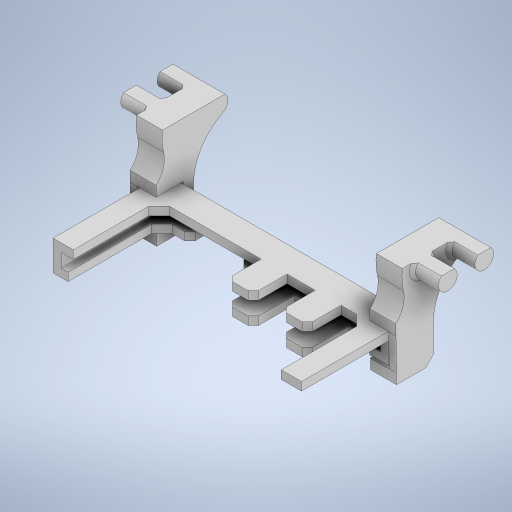
# Autodesk Inventor part: Holder-PCB
Saved by Autodesk Inventor 2024.3 (Build 283343000, 343)
## iProperties
Created: 2025-01-23
Part Number: Holder-PCB
Material: Generic
Document SubType Name: Modeling
Designer: ASUS TUF
Density: 1 g/cm^3
Appearance: Default
Author: ASUS TUF
Autodesk Inventor part; units mm, degrees
ref_plane "YZ Plane" through (0, 0, 0) normal (1, 0, 0) x (0, 1, 0)
ref_plane "XZ Plane" through (0, 0, 0) normal (0, 1, 0) x (-1, 0, 0)
ref_plane "XY Plane" through (0, 0, 0) normal (0, 0, 1) x (1, 0, 0)
sketch "Sketch1" plane through (0, 0, 0) normal (0, 0, 1) x (1, 0, 0)
  line L0 (22, 1) -> (22, -1) construction
  line L1 (-22, -1) -> (22, -1) construction
  line L2 (-22, 1) -> (-22, -1) construction
  line L3 (22, 1) -> (-22, 1) construction
  line L4 (22.3, -1.3) -> (22.3, 1.3)
  line L5 (22.3, 1.3) -> (-22.3, 1.3)
  line L6 (-22.3, 1.3) -> (-22.3, -1.3)
  line L7 (-22.3, -1.3) -> (22.3, -1.3)
  line L8 (-20, -1) -> (-20, -4.5) construction
  line L9 (23.9, -2.9) -> (23.9, 2.9)
  line L10 (23.9, 2.9) -> (-23.9, 2.9)
  line L11 (-23.9, 2.9) -> (-23.9, -2.9)
  line L12 (-23.9, -2.9) -> (23.9, -2.9)
  line L13 (-21, -2.9) -> (-21, 2.9)
  line L14 (0, -2.9) -> (0, 2.9) construction
  line L15 (21, -2.9) -> (21, 2.9)
  point P0 (0, 0)
  point P1 (21, -1.3)
  point P2 (21, 1.3)
  point P3 (-21, 1.3)
  point P4 (-21, -1.3)
  dimension "d2" = 0.3
  dimension "d3" = 1.6
  dimension "d4" = 1
  constraints: 22 end point, 2 midpoint, 2 point on line, 2 symmetric about line, 1 perpendicular, 6 other
  measures "d2" distance between parallel lines of L1 L7
  measures "d3" distance between parallel lines of L7 L12
  measures "d4" distance between parallel lines of L8 L13
extrude "Extrusion1" add sketch "Sketch1" along normal mid plane 1.5
sketch "Sketch2" plane through (0, 0, 0.75) normal (0, 0, 1) x (1, 0, 0)
  line L0 (22, 1) -> (22, -1) construction
  line L1 (-22, -1) -> (22, -1) construction
  line L2 (-22, 1) -> (-22, -1) construction
  line L3 (22, 1) -> (-22, 1) construction
  line L4 (-20, -1) -> (-20, -4.5) construction
  line L5 (23.9, -2.9) -> (-23.9, -2.9) projected
  line L6 (-23.9, -2.9) -> (-23.9, 2.9) projected
  line L7 (-23.9, 2.9) -> (23.9, 2.9) projected
  line L8 (23.9, 2.9) -> (23.9, -2.9) projected
  line L9 (22.3, -1.3) -> (22.3, 1.3)
  line L10 (22.3, 1.3) -> (-22.3, 1.3)
  line L11 (-22.3, 1.3) -> (-22.3, -1.3)
  line L12 (-22.3, -1.3) -> (22.3, -1.3)
  line L13 (-21, -2.9) -> (-21, -1.3)
  line L14 (0, -2.9) -> (0, 2.9) construction
  line L15 (-20, 1.3) -> (-20, 2.9)
  line L16 (21, -2.9) -> (21, -1.3)
  line L17 (20, 1.3) -> (20, 2.9)
  point P0 (0, 0)
  point P1 (-21, 1.3)
  dimension "d5" = 0.3
  dimension "d6" = 1
  dimension "d9" = 2
  constraints: 18 end point, 4 point on line, 4 symmetric about line, 2 midpoint, 2 perpendicular, 3 other
  measures "d5" distance between parallel lines of L1 L12
  measures "d6" distance between parallel lines of L4 L13
  measures "d9" distance between parallel lines of L2 L15
extrude "Extrusion2" add sketch "Sketch2" along normal blind 20 contours L5 L16 L12 L9 L10 L17 L7 L8 | L5 L6 L7 L15 L10 L11 L12 L13
sketch "Sketch3" plane through (0, 0, 0.75) normal (0, 0, 1) x (1, 0, 0)
  line L0 (-20, 2.9) -> (-20, 1.3)
  line L1 (-20, 1.3) -> (-22.3, 1.3)
  line L2 (-22.3, 1.3) -> (-22.3, -1.3)
  line L3 (-22.3, -1.3) -> (-21, -1.3)
  line L4 (-21, -1.3) -> (-21, -2.9)
  line L5 (-21, -2.9) -> (21, -2.9)
  line L6 (21, -2.9) -> (21, -1.3)
  line L7 (21, -1.3) -> (22.3, -1.3)
  line L8 (22.3, -1.3) -> (22.3, 1.3)
  line L9 (22.3, 1.3) -> (20, 1.3)
  line L10 (20, 1.3) -> (20, 2.9)
  line L11 (20, 2.9) -> (-20, 2.9)
  line L12 (-20, 1.3) -> (20, 1.3)
  line L13 (21, -1.3) -> (-21, -1.3)
  line L14 (-0.881943, -1.696277) -> (-0.881943, -10.1) construction
  line L15 (5.118057, -10.8) -> (5.118057, -1) construction
  line L16 (-0.381943, -2.9) -> (-0.381943, 2.9)
  line L17 (4.618057, 2.9) -> (4.618057, -2.9)
  line L18 (20, 2.9) -> (-20, 2.9)
  line L19 (9.518057, -1.696277) -> (9.518057, -10.1) construction
  line L20 (15.518057, -0.5) -> (15.518057, -6.5) construction
  line L21 (10.018057, 2.9) -> (10.018057, -2.9)
  line L22 (-21, -2.9) -> (21, -2.9)
  line L23 (15.018057, 2.9) -> (15.018057, -2.9)
  point P0 (0, 0)
  point P1 (15.018057, 1.3)
  point P2 (10.018057, 1.3)
  point P3 (4.618057, 1.3)
  point P4 (-0.381943, 1.3)
  point P5 (15.018057, -1.3)
  point P6 (10.018057, -1.3)
  point P7 (4.618057, -1.3)
  point P8 (-0.381943, -1.3)
  dimension "d21" = 0.5
  dimension "d22" = 0.5
  dimension "d23" = 0.5
  dimension "d24" = 0.5
  constraints: 20 end point, 8 point on line, 5 perpendicular, 4 vertical, 1 horizontal, 1 parallel, 8 other
  measures "d21" distance between parallel lines of L14 L16
  measures "d22" distance between parallel lines of L15 L17
  measures "d23" distance between parallel lines of L20 L23
  measures "d24" distance between parallel lines of L19 L21
extrude "Extrusion3" add sketch "Sketch3" along normal blind 3.5 contours L11 L16 L12 L0 | L11 L17 L12 L16 | L11 L21 L12 L17 | L11 L23 L12 L21 | L11 L10 L12 L23
extrude "Extrusion4" add sketch "Sketch3" along normal blind 2 contours L16 L5 L4 L13 | L13 L17 L5 L16 | L13 L21 L5 L17 | L13 L23 L5 L21 | L13 L6 L5 L23
chamfer "Chamfer1" distance 2 angle 45 4 edges at (-21, -2.1, 2.75) (-20, 2.1, 4.25) (20, 2.1, 4.25) (21, -2.1, 2.75)
sketch "Sketch4" plane through (-23.9, -2.9, -0.75) normal (0, -1, 0) x (1, 0, 0)
  line L0 (9.318057, -1.3) -> (11.268057, -1.3) construction
  line L1 (11.268057, -1.3) -> (11.268057, 2.4) construction
  line L2 (11.268057, 2.4) -> (14.768057, 2.4) construction
  line L3 (14.768057, 2.4) -> (14.768057, -1.3) construction
  line L4 (14.768057, -1.3) -> (16.718057, -1.3) construction
  line L5 (16.718057, -1.3) -> (16.718057, 6) construction
  line L6 (16.718057, 6) -> (9.318057, 6) construction
  line L7 (9.318057, 6) -> (9.318057, -1.3) construction
  line L8 (46.718057, 5.7) -> (46.718057, 7.65) construction
  line L9 (46.718057, 7.65) -> (43.018057, 7.65) construction
  line L10 (43.018057, 7.65) -> (43.018057, 11.15) construction
  line L11 (43.018057, 11.15) -> (46.718057, 11.15) construction
  line L12 (46.718057, 11.15) -> (46.718057, 13.1) construction
  line L13 (46.718057, 13.1) -> (39.418057, 13.1) construction
  line L14 (39.418057, 13.1) -> (39.418057, 5.7) construction
  line L15 (39.418057, 5.7) -> (46.718057, 5.7) construction
  line L16 (17.718057, 7) -> (17.718057, -2.3)
  line L17 (17.718057, -2.3) -> (13.768057, -2.3)
  line L18 (13.768057, -2.3) -> (13.768057, 1.4)
  line L19 (13.768057, 1.4) -> (12.268057, 1.4)
  line L20 (12.268057, 1.4) -> (12.268057, -2.3)
  line L21 (12.268057, -2.3) -> (8.318057, -2.3)
  line L22 (8.318057, -2.3) -> (8.318057, 7)
  line L23 (8.318057, 7) -> (17.718057, 7)
  line L24 (47.718057, 4.7) -> (47.718057, 8.65)
  line L25 (47.718057, 8.65) -> (44.018057, 8.65)
  line L26 (44.018057, 8.65) -> (44.018057, 10.15)
  line L27 (44.018057, 10.15) -> (47.718057, 10.15)
  line L28 (47.718057, 10.15) -> (47.718057, 14.1)
  line L29 (47.718057, 14.1) -> (38.418057, 14.1)
  line L30 (38.418057, 14.1) -> (38.418057, 4.7)
  line L31 (38.418057, 4.7) -> (47.718057, 4.7)
  line L32 (47.8, 0) -> (47.8, 21.5)
  line L33 (44.9, 21.5) -> (47.8, 21.5)
  line L34 (44.9, 5.5) -> (44.9, 21.5)
  line L35 (42.9, 3.5) -> (44.9, 5.5)
  line L36 (4.9, 3.5) -> (42.9, 3.5)
  line L37 (2.9, 5.5) -> (4.9, 3.5)
  line L38 (2.9, 5.5) -> (2.9, 21.5)
  line L39 (0, 21.5) -> (2.9, 21.5)
  line L40 (0, 21.5) -> (0, 0)
  line L41 (47.8, 0) -> (0, 0)
  line L42 (47.718057, 4.7) -> (47.8, 4.7)
  line L43 (47.718057, 14.1) -> (47.8, 14.1)
  point P0 (23.9, 0.75)
  point P1 (17.718057, 0)
  point P2 (17.718057, 3.5)
  point P3 (8.318057, 3.5)
  point P4 (8.318057, 0)
  point P5 (44.9, 14.1)
  point P6 (44.1, 4.7)
  dimension "d17" = 1
  dimension "d18" = 1
  constraints: 36 end point, 2 perpendicular, 2 point on line, 14 other
  measures "d17" distance between parallel lines of L5 L16
  measures "d18" distance between parallel lines of L15 L31
extrude "Extrusion5" cut sketch "Sketch4" against normal up to surface (4.2 mm away) contours L16 L41 L18 L19 L20 L22 L36 | L41 L20 L19 L18 | L35 L34 L25 L24 L31 | L42 L24 L25 L34 L27 L28 L43 L32 | L43 L29 L34 L33 L32 | L28 L27 L34 L29
extrude "Extrusion6" add sketch "Sketch3" along normal blind 8 from surface at 2 contours L11 L17 L12 L16 | L13 L17 L5 L16 | L11 L23 L12 L21 | L13 L23 L5 L21
chamfer "Chamfer2" distance 1 angle 45 10 edges at (4.6181, 2.1, 10.75) (4.6181, -2.1, 10.75) (-0.3819, 2.1, 10.75) (-0.3819, -2.1, 10.75) (10.0181, 2.1, 10.75) (10.0181, -2.1, 10.75) (15.0181, 2.1, 10.75) (15.0181, -2.1, 10.75) (-6.1819, -2.1, 2.75) (-15.5819, -2.1, 2.75)
ref_plane "Work Plane1" through (25.567949, 17.21409, -10.739318) normal (-1, 0, 0) x (0, 0, -1)
sketch "Sketch5" plane through (25.567949, 17.21409, -10.739318) normal (-1, 0, 0) x (0, 0, -1)
  arc A0 (-1.677124, 3.328427) -> (-4.322876, 3.328427) centre (-3, 4.828427) ccw
  line L0 (-1.677124, 3.328427) -> (-4.322876, 3.328427)
  arc A1 (-9.608071, 10.950914) -> (-8.094331, 12.258046) centre (-9.829369, 12.737259) ccw
  arc A2 (-7.504205, 12.629939) -> (-8.094331, 12.258046) centre (-3, 4.828427) ccw
  arc A3 (-5.970033, 8.970542) -> (-7.504205, 12.629939) centre (-6.504205, 10.897888) ccw
  arc A4 (-5.970033, 8.970542) -> (-6.678281, 8.227605) centre (-5.702948, 8.006869) ccw
  arc A5 (-6.678281, 8.227605) -> (-7.782915, 6.314323) centre (-3, 4.828427) ccw
  arc A6 (-7.782915, 6.314323) -> (-8.072193, 5.329494) centre (-7.104086, 5.580027) ccw
  arc A7 (-8.685534, 3.328427) -> (-8.072193, 5.329494) centre (-10.008409, 4.828427) ccw
  line L1 (-8.685534, 3.328427) -> (-11.331285, 3.328427)
  arc A8 (-11.721843, 5.860001) -> (-11.331285, 3.328427) centre (-10.008409, 4.828427) ccw
  arc A9 (-11.721843, 5.860001) -> (-11.606264, 7.489941) centre (-13.263933, 6.788418) ccw
  arc A10 (-9.608071, 10.950914) -> (-11.606264, 7.489941) centre (-3, 4.828427) ccw
  line L2 (0, 17.361989) -> (0, 0)
  line L3 (-15, 17.361989) -> (0, 17.361989)
  line L4 (-15, 0) -> (-15, 17.361989)
  line L5 (0, 0) -> (-15, 0)
  circle A11 centre (-10.008409, 4.828427) radius 1.8
  circle A12 centre (-3, 4.828427) radius 1.8
  line L6 (-11.253399, 3.528427) -> (-1.75501, 3.528427)
  point P0 (-10.739318, 17.21409)
  point P1 (-4.24499, 3.528427)
  point P2 (-8.763419, 3.528427)
  dimension "d30" = 0.2
  dimension "d31" = 0.2
  dimension "d32" = 0.2
  constraints: 2 coincident, 2 end point, 1 parallel, 6 other
  measures "d32" distance between parallel lines of L1 L6
extrude "Extrusion7" add sketch "Sketch5" along normal blind 5 and the other way blind 5 separate body contours A12 L6 | A11 L6
sketch "Sketch6" plane through (25.567949, 17.21409, -10.739318) normal (-1, 0, 0) x (0, 0, -1)
  arc A0 (-8.763419, 3.528427) -> (-11.253399, 3.528427) centre (-10.008409, 4.828427) ccw
  line L0 (-11.253399, 3.528427) -> (-8.763419, 3.528427)
  arc A1 (-1.75501, 3.528427) -> (-4.24499, 3.528427) centre (-3, 4.828427) ccw
  line L1 (-4.24499, 3.528427) -> (-1.75501, 3.528427)
  line L2 (-1.75501, 3.528427) -> (-13.75501, 3.528427)
  line L3 (-1.2, 4.828427) -> (-1.2, 12.228194) construction
  line L4 (-2.1, 6.387273) -> (-11.351496, 11.728627)
  arc A2 (-11.351496, 11.728627) -> (-13.75501, 3.528427) centre (-3, 4.828427) ccw
  line L5 (-8.763419, 3.528427) -> (-11.253399, 3.528427)
  line L6 (-1.75501, 3.528427) -> (-4.24499, 3.528427)
  point P0 (-10.739318, 17.21409)
  point P1 (-4.24499, 3.528427)
  dimension "d37" = 60
  dimension "d38" = 12
  constraints: 10 end point, 8 point on circle, 3 centre point, 2 collinear, 2 tangent, 1 coincident, 1 point on line, 1 vertical, 2 other
  measures "d37" angle of L3 L4
  measures "d38" distance of L1.end L2.end
extrude "Extrusion8" add sketch "Sketch6" along normal blind 5 contours A0 L2 A2 L4 A1 bodies 2
chamfer "Chamfer3" distance 0.6 angle 45 2 edges at (25.5679, 10.5857, -0.7309) (25.5679, 11.3054, -6.2995)
sketch "Sketch7" plane through (25.567949, 17.21409, -10.739318) normal (-1, 0, 0) x (0, 0, -1)
  line L0 (-9.989318, 14.31409) -> (-31.489318, 14.31409)
  line L1 (-31.489318, 15.91409) -> (-31.489318, 14.31409)
  line L2 (-31.489318, 15.91409) -> (-14.689318, 15.91409)
  line L3 (-14.689318, 15.91409) -> (-14.689318, 20.11409)
  line L4 (-9.989318, 20.11409) -> (-14.689318, 20.11409)
  line L5 (-9.989318, 14.31409) -> (-9.989318, 20.11409)
  line L6 (-31.689318, 14.11409) -> (-9.789318, 14.11409)
  line L7 (-9.789318, 14.11409) -> (-9.789318, 20.31409)
  line L8 (-9.789318, 20.31409) -> (-14.889318, 20.31409)
  line L9 (-14.889318, 20.31409) -> (-14.889318, 16.11409)
  line L10 (-14.889318, 16.11409) -> (-31.689318, 16.11409)
  line L11 (-31.689318, 16.11409) -> (-31.689318, 14.11409)
  arc A0 (-1.75501, 3.528427) -> (-2.1, 6.387273) centre (-3, 4.828427) ccw
  line L12 (-2.1, 6.387273) -> (-11.351496, 11.728627)
  arc A1 (-11.351496, 11.728627) -> (-13.75501, 3.528427) centre (-3, 4.828427) ccw
  line L13 (-13.75501, 3.528427) -> (-1.75501, 3.528427)
  line L14 (-16.889318, 22.31409) -> (-7.789318, 22.31409)
  line L15 (-7.789318, 22.31409) -> (-7.789318, 12.11409)
  line L16 (-7.789318, 12.11409) -> (-33.689318, 12.11409)
  line L17 (-33.689318, 12.11409) -> (-33.689318, 18.11409)
  line L18 (-33.689318, 18.11409) -> (-16.889318, 18.11409)
  line L19 (-16.889318, 18.11409) -> (-16.889318, 22.31409)
  arc A2 (-13.543372, 7.317912) -> (-14.989318, 12.11409) centre (-18.409562, 8.46691) ccw
  arc A3 (-7.789318, 15.445505) -> (-2.789318, 6.785251) centre (2.210682, 15.445505) ccw
  line L20 (-14.989318, 12.11409) -> (-14.989318, 14.11409)
  line L21 (-14.889318, 20.31409) -> (-14.889318, 22.31409)
  point P0 (-10.739318, 17.21409)
  point P1 (-14.989318, 14.31409)
  dimension "d44" = 0.2
  dimension "d46" = 2
  dimension "d47" = 5
  dimension "d48" = 10
  constraints: 28 end point, 5 point on circle, 5 point on line, 3 tangent, 2 centre point, 2 perpendicular, 1 vertical alignment, 10 other
  measures "d44" distance between parallel lines of L0 L6
  measures "d46" distance between parallel lines of L8 L14
  measures "d47" radius of A2
  measures "d48" radius of A3
extrude "Extrusion9" add sketch "Sketch7" along normal blind 5 contours L6 L7 L8 L21 L14 L15 L16 L20 | L16 L15 A3 L12 A1 A2 bodies 2
chamfer "Chamfer4" distance 1.5 angle 45 1 edges at (23.0679, -5.1, -2.95)
sketch "Sketch8" plane through (25.567949, 17.21409, -10.739318) normal (1, 0, 0) x (0, 0, -1)
  line L0 (-7.789318, -20.81409) -> (-9.289318, -22.31409)
  line L1 (-7.789318, -15.445505) -> (-7.789318, -20.81409)
  arc A0 (-2.789318, -6.785251) -> (-7.789318, -15.445505) centre (2.210682, -15.445505) ccw
  line L2 (-3.474773, -7.180998) -> (-2.789318, -6.785251)
  arc A1 (-5.017424, -3.528427) -> (-3.474773, -7.180998) centre (-3, -4.828427) ccw
  line L3 (-7.990985, -3.528427) -> (-5.017424, -3.528427)
  arc A2 (-12.025834, -3.528427) -> (-7.990985, -3.528427) centre (-10.008409, -4.828427) ccw
  line L4 (-13.75501, -3.528427) -> (-12.025834, -3.528427)
  arc A3 (-13.75501, -3.528427) -> (-13.543372, -7.317912) centre (-3, -4.828427) ccw
  arc A4 (-14.989318, -12.11409) -> (-13.543372, -7.317912) centre (-18.409562, -8.46691) ccw
  line L5 (-14.989318, -14.11409) -> (-14.989318, -12.11409)
  line L6 (-9.789318, -14.11409) -> (-14.989318, -14.11409)
  line L7 (-9.789318, -20.31409) -> (-9.789318, -14.11409)
  line L8 (-14.889318, -20.31409) -> (-9.789318, -20.31409)
  line L9 (-14.889318, -22.31409) -> (-14.889318, -20.31409)
  line L10 (-9.289318, -22.31409) -> (-14.889318, -22.31409)
  line L11 (-14.889318, -20.31409) -> (-14.989318, -14.11409)
  point P0 (-10.739318, -17.21409)
  constraints: 2 end point
extrude "Extrusion10" add sketch "Sketch8" against normal blind 1.4 contours L11 L6 L7 L8 bodies 2
mirror "Mirror1" about plane through (0, 0, 0) normal (1, 0, 0) bodies 2 separate body
body "Solid1"
body "Solid2"
body "Solid3"
